Autodesk Inventor part; units mm, degrees
(part 2 of 3)
sketch "Эскиз5" plane through (0, 2, 0) normal (0, 1, 0) x (1, 0, 0)
  line L0 (-76.014, 34.2947) -> (-34.2947, 76.014) construction
  arc A0 (-34.2947, 76.014) -> (-34.2947, 83.085) centre (-37.8302, 79.5495) ccw construction
  line L1 (-34.2947, 83.085) -> (-38.3892, 87.1795) construction
  arc A1 (-37.7453, 90.4395) -> (-38.3892, 87.1795) centre (-36.975, 88.5938) ccw construction
  arc A2 (37.7453, 90.4395) -> (-37.7453, 90.4395) centre (0, 0) ccw construction
  arc A3 (38.3892, 87.1795) -> (37.7453, 90.4395) centre (36.975, 88.5938) ccw construction
  line L2 (38.3892, 87.1795) -> (34.2947, 83.085) construction
  arc A4 (34.2947, 83.085) -> (34.2947, 76.014) centre (37.8302, 79.5495) ccw construction
  line L3 (34.2947, 76.014) -> (76.014, 34.2947) construction
  arc A5 (48.6481, 93.0503) -> (-48.6481, 93.0503) centre (0, 0) ccw construction
  arc A6 (-48.6481, 93.0503) -> (-49.3795, 88.2704) centre (-47.2582, 90.3917) ccw construction
  line L4 (-49.3795, 88.2704) -> (-46.3155, 85.2064) construction
  arc A7 (-46.3155, 73.8927) -> (-46.3155, 85.2064) centre (-51.9723, 79.5495) ccw construction
  line L5 (-46.3155, 73.8927) -> (-73.8927, 46.3155) construction
  arc A8 (-85.2064, 46.3155) -> (-73.8927, 46.3155) centre (-79.5495, 51.9723) ccw construction
  line L6 (-85.2064, 46.3155) -> (-88.2704, 49.3795) construction
  arc A9 (-88.2704, 49.3795) -> (-93.0503, 48.6481) centre (-90.3917, 47.2582) ccw construction
  arc A10 (-93.0503, 48.6481) -> (-93.0503, -48.6481) centre (0, 0) ccw construction
  arc A11 (-93.0503, -48.6481) -> (-88.2704, -49.3795) centre (-90.3917, -47.2582) ccw construction
  line L7 (-88.2704, -49.3795) -> (-85.2064, -46.3155) construction
  arc A12 (-73.8927, -46.3155) -> (-85.2064, -46.3155) centre (-79.5495, -51.9723) ccw construction
  line L8 (-73.8927, -46.3155) -> (-46.3155, -73.8927) construction
  arc A13 (-46.3155, -85.2064) -> (-46.3155, -73.8927) centre (-51.9723, -79.5495) ccw construction
  line L9 (-46.3155, -85.2064) -> (-49.3795, -88.2704) construction
  arc A14 (-49.3795, -88.2704) -> (-48.6481, -93.0503) centre (-47.2582, -90.3917) ccw construction
  arc A15 (-48.6481, -93.0503) -> (-45.42, -94.668) centre (0, 0) ccw construction
  arc A16 (-45.42, -94.668) -> (-43.0355, -94.1655) centre (-44.5548, -92.8648) ccw construction
  line L10 (-43.0355, -94.1655) -> (-18.3802, -65.3664) construction
  arc A17 (-17.477, -64.7643) -> (-18.3802, -65.3664) centre (-16.8609, -66.6671) ccw construction
  line L11 (-17.477, -64.7643) -> (-0.6161, -59.3045) construction
  arc A18 (0.6161, -59.3045) -> (-0.6161, -59.3045) centre (0, -61.2072) ccw construction
  line L12 (0.6161, -59.3045) -> (17.477, -64.7643) construction
  arc A19 (18.3802, -65.3664) -> (17.477, -64.7643) centre (16.8609, -66.6671) ccw construction
  line L13 (18.3802, -65.3664) -> (43.0355, -94.1655) construction
  arc A20 (43.0355, -94.1655) -> (45.42, -94.668) centre (44.5548, -92.8648) ccw construction
  arc A21 (45.42, -94.668) -> (48.6481, -93.0503) centre (0, 0) ccw construction
  arc A22 (48.6481, -93.0503) -> (49.3795, -88.2704) centre (47.2582, -90.3917) ccw construction
  line L14 (49.3795, -88.2704) -> (46.3155, -85.2064) construction
  arc A23 (46.3155, -73.8927) -> (46.3155, -85.2064) centre (51.9723, -79.5495) ccw construction
  line L15 (46.3155, -73.8927) -> (73.8927, -46.3155) construction
  arc A24 (85.2064, -46.3155) -> (73.8927, -46.3155) centre (79.5495, -51.9723) ccw construction
  line L16 (85.2064, -46.3155) -> (88.2704, -49.3795) construction
  arc A25 (88.2704, -49.3795) -> (93.0503, -48.6481) centre (90.3917, -47.2582) ccw construction
  arc A26 (93.0503, -48.6481) -> (93.0503, 48.6481) centre (0, 0) ccw construction
  arc A27 (93.0503, 48.6481) -> (88.2704, 49.3795) centre (90.3917, 47.2582) ccw construction
  line L17 (88.2704, 49.3795) -> (85.2064, 46.3155) construction
  arc A28 (73.8927, 46.3155) -> (85.2064, 46.3155) centre (79.5495, 51.9723) ccw construction
  line L18 (73.8927, 46.3155) -> (46.3155, 73.8927) construction
  arc A29 (46.3155, 85.2064) -> (46.3155, 73.8927) centre (51.9723, 79.5495) ccw construction
  line L19 (46.3155, 85.2064) -> (49.3795, 88.2704) construction
  arc A30 (49.3795, 88.2704) -> (48.6481, 93.0503) centre (47.2582, 90.3917) ccw construction
  arc A31 (76.014, 34.2947) -> (83.085, 34.2947) centre (79.5495, 37.8302) ccw construction
  line L20 (83.085, 34.2947) -> (87.1795, 38.3892) construction
  arc A32 (90.4395, 37.7453) -> (87.1795, 38.3892) centre (88.5938, 36.975) ccw construction
  arc A33 (90.4395, -37.7453) -> (90.4395, 37.7453) centre (0, 0) ccw construction
  arc A34 (87.1795, -38.3892) -> (90.4395, -37.7453) centre (88.5938, -36.975) ccw construction
  line L21 (87.1795, -38.3892) -> (83.085, -34.2947) construction
  arc A35 (83.085, -34.2947) -> (76.014, -34.2947) centre (79.5495, -37.8302) ccw construction
  line L22 (76.014, -34.2947) -> (37.1244, -73.1843) construction
  line L23 (-37.1244, -73.1843) -> (-76.014, -34.2947) construction
  arc A36 (-76.014, -34.2947) -> (-83.085, -34.2947) centre (-79.5495, -37.8302) ccw construction
  line L24 (-83.085, -34.2947) -> (-87.1795, -38.3892) construction
  arc A37 (-90.4395, -37.7453) -> (-87.1795, -38.3892) centre (-88.5938, -36.975) ccw construction
  arc A38 (-90.4395, 37.7453) -> (-90.4395, -37.7453) centre (0, 0) ccw construction
  arc A39 (-87.1795, 38.3892) -> (-90.4395, 37.7453) centre (-88.5938, 36.975) ccw construction
  line L25 (-87.1795, 38.3892) -> (-83.085, 34.2947) construction
  arc A40 (-83.085, 34.2947) -> (-76.014, 34.2947) centre (-79.5495, 37.8302) ccw construction
  arc A41 (34.1909, -73.0707) -> (37.1244, -73.1843) centre (35.7102, -71.7701) ccw construction
  line L26 (34.1909, -73.0707) -> (25.4187, -62.8242) construction
  arc A42 (24.842, -61.8893) -> (25.4187, -62.8242) centre (28.1154, -60.5155) ccw construction
  line L27 (24.842, -61.8893) -> (23.8313, -59.4808) construction
  arc A43 (23.8313, -59.4808) -> (21.0049, -57.3328) centre (20.5578, -60.8546) ccw construction
  line L28 (21.0049, -57.3328) -> (15.1585, -56.5907) construction
  arc A44 (14.5119, -56.4463) -> (15.1585, -56.5907) centre (15.6055, -53.069) ccw construction
  line L29 (14.5119, -56.4463) -> (0.6161, -51.9466) construction
  arc A45 (0.6161, -51.9466) -> (-0.6161, -51.9466) centre (0, -53.8493) ccw construction
  line L30 (-0.6161, -51.9466) -> (-14.5119, -56.4463) construction
  arc A46 (-15.1585, -56.5907) -> (-14.5119, -56.4463) centre (-15.6055, -53.069) ccw construction
  line L31 (-15.1585, -56.5907) -> (-21.0049, -57.3328) construction
  arc A47 (-21.0049, -57.3328) -> (-23.8313, -59.4808) centre (-20.5578, -60.8546) ccw construction
  line L32 (-23.8313, -59.4808) -> (-24.842, -61.8893) construction
  arc A48 (-25.4187, -62.8242) -> (-24.842, -61.8893) centre (-28.1154, -60.5155) ccw construction
  line L33 (-25.4187, -62.8242) -> (-34.1909, -73.0707) construction
  arc A49 (-37.1244, -73.1843) -> (-34.1909, -73.0707) centre (-35.7102, -71.7701) ccw construction
  circle A50 centre (-37.8302, 79.5495) radius 1.6 construction
  circle A51 centre (-79.5495, 37.8302) radius 1.6 construction
  circle A52 centre (-79.5495, -37.8302) radius 1.6 construction
  circle A53 centre (79.5495, -37.8302) radius 1.6 construction
  circle A54 centre (37.8302, 79.5495) radius 1.6 construction
  circle A55 centre (79.5495, 37.8302) radius 1.6 construction
  circle A56 centre (-20.5578, -60.8546) radius 1.55 construction
  circle A57 centre (20.5578, -60.8546) radius 1.55 construction
  circle A58 centre (37.8302, -79.5495) radius 1.6 construction
  circle A59 centre (-37.8302, -79.5495) radius 1.6 construction
  circle A60 centre (0, -40) radius 1.6
  line L34 (0, -40.1335) -> (0, 0) construction
  arc A61 (0, -36) -> (-3.6492, -38.362) centre (0, -40) ccw
  line L35 (19.2746, -40.1335) -> (6.3862, -40.1335) construction
  line L36 (19.2746, -40.1335) -> (-19.2746, -40.1335) construction
  line L37 (-6.3862, -40.1335) -> (-19.2746, -40.1335) construction
  arc A62 (3.6492, -38.362) -> (0, -36) centre (0, -40) ccw
  arc A63 (-3.9978, -40.1335) -> (3.9978, -40.1335) centre (0, -40) ccw construction
  arc A64 (3.6492, -38.362) -> (6.3862, -40.1335) centre (6.3862, -37.1335) ccw
  arc A65 (-6.3862, -40.1335) -> (-3.6492, -38.362) centre (-6.3862, -37.1335) ccw
  line L38 (6.3862, -40.1335) -> (3.8373, -44.953)
  line L39 (3.8373, -44.953) -> (-3.2661, -45.2784)
  line L40 (-3.2661, -45.2784) -> (-6.3862, -40.1335)
  dimension "d100" = 3.2
  dimension "d101" = 40
  dimension "d103" = 3
  dimension "d104" = 4
  constraints: 12 end point, 12 point on circle, 6 centre point, 6 point on line, 4 tangent, 1 coincident, 1 equal radius, 1 vertical
  measures "d100" diameter of A60
  measures "d101" distance of point (0, 0) A60.centre
  measures "d103" radius of A64
  measures "d104" radius of A63
ref_plane "РабПлоскость8" through (0, 2, 0) normal (0, 1, 0) x (1, 0, 0)
sketch "Эскиз6" plane through (0, 2, 0) normal (0, 1, 0) x (1, 0, 0)
  line L0 (-76.014, 34.2947) -> (-34.2947, 76.014) construction
  arc A0 (-34.2947, 76.014) -> (-34.2947, 83.085) centre (-37.8302, 79.5495) ccw construction
  line L1 (-34.2947, 83.085) -> (-38.3892, 87.1795) construction
  arc A1 (-37.7453, 90.4395) -> (-38.3892, 87.1795) centre (-36.975, 88.5938) ccw construction
  arc A2 (37.7453, 90.4395) -> (-37.7453, 90.4395) centre (0, 0) ccw construction
  arc A3 (38.3892, 87.1795) -> (37.7453, 90.4395) centre (36.975, 88.5938) ccw construction
  line L2 (38.3892, 87.1795) -> (34.2947, 83.085) construction
  arc A4 (34.2947, 83.085) -> (34.2947, 76.014) centre (37.8302, 79.5495) ccw construction
  line L3 (34.2947, 76.014) -> (76.014, 34.2947) construction
  arc A5 (48.6481, 93.0503) -> (-48.6481, 93.0503) centre (0, 0) ccw construction
  arc A6 (-48.6481, 93.0503) -> (-49.3795, 88.2704) centre (-47.2582, 90.3917) ccw construction
  line L4 (-49.3795, 88.2704) -> (-46.3155, 85.2064) construction
  arc A7 (-46.3155, 73.8927) -> (-46.3155, 85.2064) centre (-51.9723, 79.5495) ccw construction
  line L5 (-46.3155, 73.8927) -> (-73.8927, 46.3155) construction
  arc A8 (-85.2064, 46.3155) -> (-73.8927, 46.3155) centre (-79.5495, 51.9723) ccw construction
  line L6 (-85.2064, 46.3155) -> (-88.2704, 49.3795) construction
  arc A9 (-88.2704, 49.3795) -> (-93.0503, 48.6481) centre (-90.3917, 47.2582) ccw construction
  arc A10 (-93.0503, 48.6481) -> (-93.0503, -48.6481) centre (0, 0) ccw construction
  arc A11 (-93.0503, -48.6481) -> (-88.2704, -49.3795) centre (-90.3917, -47.2582) ccw construction
  line L7 (-88.2704, -49.3795) -> (-85.2064, -46.3155) construction
  arc A12 (-73.8927, -46.3155) -> (-85.2064, -46.3155) centre (-79.5495, -51.9723) ccw construction
  line L8 (-73.8927, -46.3155) -> (-46.3155, -73.8927) construction
  arc A13 (-46.3155, -85.2064) -> (-46.3155, -73.8927) centre (-51.9723, -79.5495) ccw construction
  line L9 (-46.3155, -85.2064) -> (-49.3795, -88.2704) construction
  arc A14 (-49.3795, -88.2704) -> (-48.6481, -93.0503) centre (-47.2582, -90.3917) ccw construction
  arc A15 (-48.6481, -93.0503) -> (-45.42, -94.668) centre (0, 0) ccw construction
  arc A16 (-45.42, -94.668) -> (-43.0355, -94.1655) centre (-44.5548, -92.8648) ccw construction
  line L10 (-43.0355, -94.1655) -> (-18.3802, -65.3664) construction
  arc A17 (-17.477, -64.7643) -> (-18.3802, -65.3664) centre (-16.8609, -66.6671) ccw construction
  line L11 (-17.477, -64.7643) -> (-0.6161, -59.3045) construction
  arc A18 (0.6161, -59.3045) -> (-0.6161, -59.3045) centre (0, -61.2072) ccw construction
  line L12 (0.6161, -59.3045) -> (17.477, -64.7643) construction
  arc A19 (18.3802, -65.3664) -> (17.477, -64.7643) centre (16.8609, -66.6671) ccw construction
  line L13 (18.3802, -65.3664) -> (43.0355, -94.1655) construction
  arc A20 (43.0355, -94.1655) -> (45.42, -94.668) centre (44.5548, -92.8648) ccw construction
  arc A21 (45.42, -94.668) -> (48.6481, -93.0503) centre (0, 0) ccw construction
  arc A22 (48.6481, -93.0503) -> (49.3795, -88.2704) centre (47.2582, -90.3917) ccw construction
  line L14 (49.3795, -88.2704) -> (46.3155, -85.2064) construction
  arc A23 (46.3155, -73.8927) -> (46.3155, -85.2064) centre (51.9723, -79.5495) ccw construction
  line L15 (46.3155, -73.8927) -> (73.8927, -46.3155) construction
  arc A24 (85.2064, -46.3155) -> (73.8927, -46.3155) centre (79.5495, -51.9723) ccw construction
  line L16 (85.2064, -46.3155) -> (88.2704, -49.3795) construction
  arc A25 (88.2704, -49.3795) -> (93.0503, -48.6481) centre (90.3917, -47.2582) ccw construction
  arc A26 (93.0503, -48.6481) -> (93.0503, 48.6481) centre (0, 0) ccw construction
  arc A27 (93.0503, 48.6481) -> (88.2704, 49.3795) centre (90.3917, 47.2582) ccw construction
  line L17 (88.2704, 49.3795) -> (85.2064, 46.3155) construction
  arc A28 (73.8927, 46.3155) -> (85.2064, 46.3155) centre (79.5495, 51.9723) ccw construction
  line L18 (73.8927, 46.3155) -> (46.3155, 73.8927) construction
  arc A29 (46.3155, 85.2064) -> (46.3155, 73.8927) centre (51.9723, 79.5495) ccw construction
  line L19 (46.3155, 85.2064) -> (49.3795, 88.2704) construction
  arc A30 (49.3795, 88.2704) -> (48.6481, 93.0503) centre (47.2582, 90.3917) ccw construction
  arc A31 (76.014, 34.2947) -> (83.085, 34.2947) centre (79.5495, 37.8302) ccw construction
  line L20 (83.085, 34.2947) -> (87.1795, 38.3892) construction
  arc A32 (90.4395, 37.7453) -> (87.1795, 38.3892) centre (88.5938, 36.975) ccw construction
  arc A33 (90.4395, -37.7453) -> (90.4395, 37.7453) centre (0, 0) ccw construction
  arc A34 (87.1795, -38.3892) -> (90.4395, -37.7453) centre (88.5938, -36.975) ccw construction
  line L21 (87.1795, -38.3892) -> (83.085, -34.2947) construction
  arc A35 (83.085, -34.2947) -> (76.014, -34.2947) centre (79.5495, -37.8302) ccw construction
  line L22 (76.014, -34.2947) -> (37.1244, -73.1843) construction
  line L23 (-37.1244, -73.1843) -> (-76.014, -34.2947) construction
  arc A36 (-76.014, -34.2947) -> (-83.085, -34.2947) centre (-79.5495, -37.8302) ccw construction
  line L24 (-83.085, -34.2947) -> (-87.1795, -38.3892) construction
  arc A37 (-90.4395, -37.7453) -> (-87.1795, -38.3892) centre (-88.5938, -36.975) ccw construction
  arc A38 (-90.4395, 37.7453) -> (-90.4395, -37.7453) centre (0, 0) ccw construction
  arc A39 (-87.1795, 38.3892) -> (-90.4395, 37.7453) centre (-88.5938, 36.975) ccw construction
  line L25 (-87.1795, 38.3892) -> (-83.085, 34.2947) construction
  arc A40 (-83.085, 34.2947) -> (-76.014, 34.2947) centre (-79.5495, 37.8302) ccw construction
  arc A41 (34.1909, -73.0707) -> (37.1244, -73.1843) centre (35.7102, -71.7701) ccw construction
  line L26 (34.1909, -73.0707) -> (25.4187, -62.8242) construction
  arc A42 (24.842, -61.8893) -> (25.4187, -62.8242) centre (28.1154, -60.5155) ccw construction
  line L27 (24.842, -61.8893) -> (23.8313, -59.4808) construction
  arc A43 (23.8313, -59.4808) -> (21.0049, -57.3328) centre (20.5578, -60.8546) ccw construction
  line L28 (21.0049, -57.3328) -> (15.1585, -56.5907) construction
  arc A44 (14.5119, -56.4463) -> (15.1585, -56.5907) centre (15.6055, -53.069) ccw construction
  line L29 (14.5119, -56.4463) -> (0.6161, -51.9466) construction
  arc A45 (0.6161, -51.9466) -> (-0.6161, -51.9466) centre (0, -53.8493) ccw construction
  line L30 (-0.6161, -51.9466) -> (-14.5119, -56.4463) construction
  arc A46 (-15.1585, -56.5907) -> (-14.5119, -56.4463) centre (-15.6055, -53.069) ccw construction
  line L31 (-15.1585, -56.5907) -> (-21.0049, -57.3328) construction
  arc A47 (-21.0049, -57.3328) -> (-23.8313, -59.4808) centre (-20.5578, -60.8546) ccw construction
  line L32 (-23.8313, -59.4808) -> (-24.842, -61.8893) construction
  arc A48 (-25.4187, -62.8242) -> (-24.842, -61.8893) centre (-28.1154, -60.5155) ccw construction
  line L33 (-25.4187, -62.8242) -> (-34.1909, -73.0707) construction
  arc A49 (-37.1244, -73.1843) -> (-34.1909, -73.0707) centre (-35.7102, -71.7701) ccw construction
  circle A50 centre (-37.8302, 79.5495) radius 1.6 construction
  circle A51 centre (-79.5495, 37.8302) radius 1.6 construction
  circle A52 centre (-79.5495, -37.8302) radius 1.6 construction
  circle A53 centre (79.5495, -37.8302) radius 1.6 construction
  circle A54 centre (37.8302, 79.5495) radius 1.6 construction
  circle A55 centre (79.5495, 37.8302) radius 1.6 construction
  circle A56 centre (-20.5578, -60.8546) radius 1.55 construction
  circle A57 centre (20.5578, -60.8546) radius 1.55 construction
  circle A58 centre (37.8302, -79.5495) radius 1.6 construction
  circle A59 centre (-37.8302, -79.5495) radius 1.6 construction
  line L34 (0, 0) -> (0, 105) construction
  arc A60 (48.6481, 93.0503) -> (-48.6481, 93.0503) centre (0, 0) ccw construction
  line L35 (-19.5, 5.5231) -> (19.5, 5.5231) construction
  line L36 (19.5, 5.5231) -> (19.5, 136.6901) construction
  line L37 (19.5, 136.6901) -> (-19.5, 136.6901) construction
  line L38 (-19.5, 136.6901) -> (-19.5, 5.5231) construction
  circle A61 centre (-24, 98.1071) radius 4 construction
  circle A62 centre (24, 98.1071) radius 4 construction
  arc A63 (-21.3158, 95.1414) -> (20.4598, 95.3292) centre (0, 0) ccw construction
  arc A64 (-23.5, 93.6349) -> (-20.4598, 95.3292) centre (-24, 98.1071) ccw
  line L39 (-23.5, 49.663) -> (-23.5, 93.6349)
  line L40 (-20, 47.2032) -> (-20, 95.4267)
  arc A65 (-19.0919, 46.6335) -> (-21.4454, 47.6084) centre (-21.9203, 43.1335) ccw
  line L41 (-21.4454, 47.6084) -> (-23.5, 49.663)
  line L42 (-21.6698, 47.1257) -> (-42.4264, 67.8823) construction
  line L43 (-42.4264, 67.8823) -> (-34.2947, 76.014) construction
  line L44 (-19.0919, 46.6335) -> (-6.5611, 46.6335)
  arc A66 (0, 41.5) -> (3.9366, 48.1801) centre (0, 46) ccw construction
  arc A67 (-4.4552, 46.6335) -> (0, 41.5) centre (0, 46) ccw construction
  arc A68 (-6.5611, 46.6335) -> (-3.9366, 48.1801) centre (-6.5611, 49.6335) ccw
  line L45 (-23.5, 49.663) -> (-42.0729, 68.2358) construction
  arc A69 (-18.5662, 46.1335) -> (-19.0919, 46.6335) centre (-21.9203, 43.1335) ccw construction
  arc A70 (-21.4454, 47.6084) -> (-18.5662, 46.1335) centre (-21.9203, 43.1335) ccw construction
  arc A71 (-25.858, 94.0086) -> (-23.5, 93.6349) centre (-24, 98.1071) ccw construction
  arc A72 (-20.4598, 95.3292) -> (-25.858, 94.0086) centre (-24, 98.1071) ccw construction
  arc A73 (-20.4598, 95.3292) -> (-21.3158, 95.1414) centre (0, 0) ccw construction
  arc A74 (20.4598, 95.3292) -> (23.5, 93.6349) centre (24, 98.1071) ccw
  line L46 (23.5, 49.663) -> (23.5, 93.6349)
  line L47 (20, 47.2032) -> (20, 95.4267)
  arc A75 (21.4454, 47.6084) -> (19.0919, 46.6335) centre (21.9203, 43.1335) ccw
  line L48 (21.4454, 47.6084) -> (23.5, 49.663)
  line L49 (19.0919, 46.6335) -> (6.5611, 46.6335)
  arc A76 (3.9366, 48.1801) -> (6.5611, 46.6335) centre (6.5611, 49.6335) ccw
  arc A77 (3.9366, 48.1801) -> (-3.9366, 48.1801) centre (0, 46) ccw
  arc A78 (20.4598, 95.3292) -> (-20.4598, 95.3292) centre (0, 0) ccw
  circle A79 centre (0, 46) radius 1.5
  dimension "d112" = 8
  dimension "d111" = 39
  dimension "d114" = 9
  dimension "d115" = 4
  dimension "d116" = 0.5
  dimension "d117" = 9
  dimension "d118" = 0.5
  dimension "d120" = 9
  dimension "d121" = 3
  dimension "d179" = 3
  constraints: 42 point on circle, 28 end point, 18 centre point, 13 symmetric about line, 4 parallel, 3 coincident, 3 point on line, 2 horizontal, 2 tangent, 2 vertical, 1 perpendicular, 8 other
  measures "d111" distance of L37.end L36.end
  measures "d114" diameter of A64
  measures "d115" distance between parallel lines of L38 L39
  measures "d116" distance between parallel lines of L38 L40
  measures "d117" diameter of A65
  measures "d118" distance between parallel lines of L42 L41
  measures "d120" diameter of A66
  measures "d121" radius of A68
  measures "d179" diameter of A79
extrude "Выдавливание9" add sketch "Эскиз6" along normal blind 1.85 and the other way blind 2 contours A64 A78 L40 A65 L41 L39 | A78 L47 A75 L49 A76 A77 A68 L44 A65 L40 | A78 A74 L46 L48 A75 L47
extrude "Выдавливание10" add sketch "Эскиз6" along normal blind 6.85 contours A64 A78 L40 A65 L41 L39 | A78 A74 L46 L48 A75 L47
ref_plane "РабПлоскость1" through (0, 8.85, 0) normal (0, 1, 0) x (1, 0, 0)
sketch "Эскиз7" plane through (0, 8.85, 0) normal (0, 1, 0) x (1, 0, 0)
  line L0 (-20, 95.4267) -> (-20, 47.2032) projected
  arc A0 (-19.0919, 46.6335) -> (-20, 47.2032) centre (-21.9203, 43.1335) ccw projected
  line L1 (-19.0919, 46.6335) -> (-6.5611, 46.6335) projected
  arc A1 (-6.5611, 46.6335) -> (-3.9366, 48.1801) centre (-6.5611, 49.6335) ccw construction
  arc A2 (3.9366, 48.1801) -> (-3.9366, 48.1801) centre (0, 46) ccw construction
  arc A3 (3.9366, 48.1801) -> (6.5611, 46.6335) centre (6.5611, 49.6335) ccw construction
  line L2 (6.5611, 46.6335) -> (19.0919, 46.6335) projected
  arc A4 (20, 47.2032) -> (19.0919, 46.6335) centre (21.9203, 43.1335) ccw projected
  line L3 (20, 47.2032) -> (20, 95.4267) projected
  arc A5 (20, 95.4267) -> (-20, 95.4267) centre (0, 0) ccw projected
  arc A6 (-20, 95.4267) -> (-20.4598, 95.3292) centre (0, 0) ccw projected
  arc A7 (-23.5, 93.6349) -> (-20.4598, 95.3292) centre (-24, 98.1071) ccw projected
  line L4 (-23.5, 93.6349) -> (-23.5, 49.663) projected
  line L5 (-23.5, 49.663) -> (-21.4454, 47.6084) projected
  arc A8 (-20, 47.2032) -> (-21.4454, 47.6084) centre (-21.9203, 43.1335) ccw projected
  line L6 (-20, 47.2032) -> (-20, 95.4267) projected
  arc A9 (20.4598, 95.3292) -> (20, 95.4267) centre (0, 0) ccw projected
  line L7 (20, 95.4267) -> (20, 47.2032) projected
  arc A10 (21.4454, 47.6084) -> (20, 47.2032) centre (21.9203, 43.1335) ccw projected
  line L8 (21.4454, 47.6084) -> (23.5, 49.663) projected
  line L9 (23.5, 49.663) -> (23.5, 93.6349) projected
  arc A11 (20.4598, 95.3292) -> (23.5, 93.6349) centre (24, 98.1071) ccw projected
  line L10 (18.2, 46.6335) -> (18.2, 95.7863)
  arc A12 (3.5768, 47.7906) -> (-3.5768, 47.7906) centre (0, 46) ccw construction
  line L11 (0, 46) -> (0, 97.5) construction
  line L12 (-18.2, 46.6335) -> (-18.2, 95.7863)
  point P0 (-20, 95.4267)
  point P1 (-20, 47.2032)
  dimension "d129" = 1.8
  constraints: 6 end point, 2 point on circle, 2 symmetric about line, 1 point on line, 1 vertical
  measures "d129" distance between parallel lines of L3 L10
extrude "Выдавливание11" add sketch "Эскиз7" along normal blind 5
chamfer "Фаска1" distance 1.8 angle 45 2 edges at (18.2, 8.85, -71.2099) (-18.2, 8.85, -71.2099)
fillet "Сопряжение1" radius 3 2 edges at (23.5, 13.85, -71.6489) (-23.5, 13.85, -71.6489)
fillet "Сопряжение2" radius 1 2 edges at (18.2, 13.85, -71.2099) (-18.2, 13.85, -71.2099)
ref_plane "РабПлоскость2" through (6.5611, 3.85, -46.6335) normal (0, 0, 1) x (1, 0, 0)
sketch "Эскиз8" plane through (6.5611, 3.85, -46.6335) normal (0, 0, 1) x (1, 0, 0)
  line L0 (-26.5611, 0) -> (-25.6529, 0) construction
  line L1 (-25.6529, 0) -> (-13.1221, 0) construction
  line L2 (-13.1221, 0) -> (-10.4977, 0) construction
  line L3 (-10.4977, 0) -> (-2.6244, 0) construction
  line L4 (-2.6244, 0) -> (0, 0) construction
  line L5 (0, 0) -> (12.5308, 0) construction
  line L6 (12.5308, 0) -> (13.4389, 0) construction
  line L7 (13.4389, 0) -> (-26.5611, 0) construction
  line L8 (-24.7611, 6.8) -> (-24.7611, 9) construction
  line L9 (-26.5611, 5) -> (-24.7611, 6.8) construction
  line L10 (-26.5611, 0) -> (-26.5611, 5) construction
  line L11 (13.4389, 0) -> (-26.5611, 0) construction
  line L12 (13.4389, 0) -> (13.4389, 5) construction
  line L13 (11.6389, 6.8) -> (13.4389, 5) construction
  line L14 (11.6389, 6.8) -> (11.6389, 9) construction
  line L15 (13.8987, 10) -> (12.6389, 10) construction
  line L16 (13.8987, -3.85) -> (13.8987, 10) construction
  line L17 (-27.0209, -3.85) -> (13.8987, -3.85) construction
  line L18 (-27.0209, -3.85) -> (-27.0209, 10) construction
  line L19 (-25.7611, 10) -> (-27.0209, 10) construction
  line L20 (-27.0209, 10) -> (-27.0611, 10) construction
  line L21 (-27.0209, -3.85) -> (-27.0209, 10) construction
  line L22 (-30.0611, -3.85) -> (-27.0209, -3.85) construction
  line L23 (-30.0611, -3.85) -> (-30.0611, 7) construction
  line L24 (16.9389, -3.85) -> (16.9389, 7) construction
  line L25 (13.8987, -3.85) -> (16.9389, -3.85) construction
  line L26 (13.8987, -3.85) -> (13.8987, 10) construction
  line L27 (13.9389, 10) -> (13.8987, 10) construction
  line L28 (-6.5611, -3.85) -> (-6.5611, 0) construction
  line L29 (-6.5611, -1.85) -> (-6.5611, 0.15) construction
  line L30 (-8.1611, -1.85) -> (-4.9611, -1.85) construction
  line L31 (-11.4446, 0.15) -> (-1.6776, 0.15) construction
  line L32 (-6.5611, -1.85) -> (-4.0611, -1.85) construction
  line L33 (-4.0611, -1.85) -> (-1.6776, 0.15) construction
  line L34 (-6.5611, -1.85) -> (-9.0611, -1.85) construction
  line L35 (-9.0611, -1.85) -> (-11.4446, 0.15) construction
  line L36 (-11.7325, 0) -> (-9.5278, -1.85)
  line L37 (-2.9842, -1.85) -> (-10.1379, -1.85) construction
  line L38 (-1.3896, 0) -> (-3.5943, -1.85)
  line L39 (-1.3896, 0) -> (-11.7325, 0)
  line L40 (13.4389, 0) -> (-26.5611, 0) projected
  line L41 (-9.5278, -1.85) -> (-3.5943, -1.85)
  dimension "d138" = 2
  dimension "d139" = 2.5
  dimension "d141" = 40
  dimension "d142" = 0.3
  constraints: 22 end point, 5 point on line, 4 symmetric about line, 3 midpoint, 2 collinear, 2 parallel, 1 horizontal, 5 other
  measures "d138" distance of L29.start L29.end
  measures "d139" distance of L29.start L32.end
  measures "d141" angle of L31 L33
  measures "d142" distance between parallel lines of L35 L36
extrude "Выдавливание12" cut sketch "Эскиз8" against normal mid plane 300
ref_plane "РабПлоскость9" through (0, 2, 0) normal (0, 1, 0) x (1, 0, 0)
sketch "Эскиз9" plane through (0, 2, 0) normal (0, 1, 0) x (1, 0, 0)
  line L0 (-20, 95.4267) -> (-20, 47.2032) construction
  line L1 (-20, 47.2032) -> (-20, 95.4267) construction
  line L2 (63.6396, 46.669) -> (43.8406, 26.8701) construction
  line L3 (20, 47.2032) -> (20, 95.4267) construction
  line L4 (20, 95.4267) -> (20, 47.2032) construction
  circle A0 centre (-24, 98.1071) radius 1.6 construction
  arc A1 (-25.8102, 94.5401) -> (-20.7476, 95.7786) centre (-24, 98.1071) ccw construction
  circle A2 centre (24, 98.1071) radius 1.6 construction
  arc A3 (20.7476, 95.7786) -> (25.8102, 94.5401) centre (24, 98.1071) ccw construction
  arc A4 (-27.022, 95.4865) -> (-25, 94.2341) centre (-24, 98.1071) ccw
  line L5 (-34.2947, 83.085) -> (-38.3892, 87.1795) construction
  line L6 (76.014, -34.2947) -> (37.1244, -73.1843) construction
  arc A5 (34.1909, -73.0707) -> (37.1244, -73.1843) centre (35.7102, -71.7701) ccw construction
  line L7 (34.1909, -73.0707) -> (25.4187, -62.8242) construction
  arc A6 (24.842, -61.8893) -> (25.4187, -62.8242) centre (28.1154, -60.5155) ccw construction
  line L8 (24.842, -61.8893) -> (23.8313, -59.4808) construction
  arc A7 (23.8313, -59.4808) -> (21.0049, -57.3328) centre (20.5578, -60.8546) ccw construction
  line L9 (21.0049, -57.3328) -> (15.1585, -56.5907) construction
  arc A8 (14.5119, -56.4463) -> (15.1585, -56.5907) centre (15.6055, -53.069) ccw construction
  line L10 (14.5119, -56.4463) -> (0.6161, -51.9466) construction
  arc A9 (0.6161, -51.9466) -> (-0.6161, -51.9466) centre (0, -53.8493) ccw construction
  line L11 (-0.6161, -51.9466) -> (-14.5119, -56.4463) construction
  arc A10 (-15.1585, -56.5907) -> (-14.5119, -56.4463) centre (-15.6055, -53.069) ccw construction
  line L12 (-15.1585, -56.5907) -> (-21.0049, -57.3328) construction
  arc A11 (-21.0049, -57.3328) -> (-23.8313, -59.4808) centre (-20.5578, -60.8546) ccw construction
  line L13 (-23.8313, -59.4808) -> (-24.842, -61.8893) construction
  arc A12 (-25.4187, -62.8242) -> (-24.842, -61.8893) centre (-28.1154, -60.5155) ccw construction
  line L14 (-25.4187, -62.8242) -> (-34.1909, -73.0707) construction
  arc A13 (-37.1244, -73.1843) -> (-34.1909, -73.0707) centre (-35.7102, -71.7701) ccw construction
  line L15 (-37.1244, -73.1843) -> (-76.014, -34.2947) construction
  line L16 (-76.014, 34.2947) -> (-34.2947, 76.014) construction
  arc A14 (-34.2947, 76.014) -> (-34.2947, 83.085) centre (-37.8302, 79.5495) ccw construction
  line L17 (-34.2947, 83.085) -> (-38.3892, 87.1795) construction
  arc A15 (-37.7453, 90.4395) -> (-38.3892, 87.1795) centre (-36.975, 88.5938) ccw construction
  arc A16 (37.7453, 90.4395) -> (-37.7453, 90.4395) centre (0, 0) ccw construction
  arc A17 (38.3892, 87.1795) -> (37.7453, 90.4395) centre (36.975, 88.5938) ccw construction
  line L18 (38.3892, 87.1795) -> (34.2947, 83.085) construction
  arc A18 (34.2947, 83.085) -> (34.2947, 76.014) centre (37.8302, 79.5495) ccw construction
  line L19 (34.2947, 76.014) -> (76.014, 34.2947) construction
  arc A19 (76.014, 34.2947) -> (83.085, 34.2947) centre (79.5495, 37.8302) ccw construction
  line L20 (83.085, 34.2947) -> (87.1795, 38.3892) construction
  arc A20 (90.4395, 37.7453) -> (87.1795, 38.3892) centre (88.5938, 36.975) ccw construction
  arc A21 (90.4395, -37.7453) -> (90.4395, 37.7453) centre (0, 0) ccw construction
  arc A22 (87.1795, -38.3892) -> (90.4395, -37.7453) centre (88.5938, -36.975) ccw construction
  line L21 (87.1795, -38.3892) -> (83.085, -34.2947) construction
  arc A23 (83.085, -34.2947) -> (76.014, -34.2947) centre (79.5495, -37.8302) ccw construction
  circle A24 centre (79.5495, -37.8302) radius 1.6 construction
  circle A25 centre (37.8302, 79.5495) radius 1.6 construction
  circle A26 centre (79.5495, 37.8302) radius 1.6 construction
  circle A27 centre (20.5578, -60.8546) radius 1.55 construction
  circle A28 centre (37.8302, -79.5495) radius 1.6 construction
  arc A29 (48.6481, 93.0503) -> (-48.6481, 93.0503) centre (0, 0) ccw construction
  arc A30 (-48.6481, 93.0503) -> (-49.3795, 88.2704) centre (-47.2582, 90.3917) ccw construction
  line L22 (-49.3795, 88.2704) -> (-46.3155, 85.2064) construction
  arc A31 (-46.3155, 73.8927) -> (-46.3155, 85.2064) centre (-51.9723, 79.5495) ccw construction
  line L23 (-46.3155, 73.8927) -> (-73.8927, 46.3155) construction
  arc A32 (-85.2064, 46.3155) -> (-73.8927, 46.3155) centre (-79.5495, 51.9723) ccw construction
  line L24 (-85.2064, 46.3155) -> (-88.2704, 49.3795) construction
  arc A33 (-88.2704, 49.3795) -> (-93.0503, 48.6481) centre (-90.3917, 47.2582) ccw construction
  arc A34 (-93.0503, 48.6481) -> (-93.0503, -48.6481) centre (0, 0) ccw construction
  arc A35 (-93.0503, -48.6481) -> (-88.2704, -49.3795) centre (-90.3917, -47.2582) ccw construction
  line L25 (-88.2704, -49.3795) -> (-85.2064, -46.3155) construction
  arc A36 (-73.8927, -46.3155) -> (-85.2064, -46.3155) centre (-79.5495, -51.9723) ccw construction
  line L26 (-73.8927, -46.3155) -> (-46.3155, -73.8927) construction
  arc A37 (-46.3155, -85.2064) -> (-46.3155, -73.8927) centre (-51.9723, -79.5495) ccw construction
  line L27 (-46.3155, -85.2064) -> (-49.3795, -88.2704) construction
  arc A38 (-49.3795, -88.2704) -> (-48.6481, -93.0503) centre (-47.2582, -90.3917) ccw construction
  arc A39 (-48.6481, -93.0503) -> (-45.42, -94.668) centre (0, 0) ccw construction
  arc A40 (-45.42, -94.668) -> (-43.0355, -94.1655) centre (-44.5548, -92.8648) ccw construction
  line L28 (-43.0355, -94.1655) -> (-18.3802, -65.3664) construction
  arc A41 (-17.477, -64.7643) -> (-18.3802, -65.3664) centre (-16.8609, -66.6671) ccw construction
  line L29 (-17.477, -64.7643) -> (-0.6161, -59.3045) construction
  arc A42 (0.6161, -59.3045) -> (-0.6161, -59.3045) centre (0, -61.2072) ccw construction
  line L30 (0.6161, -59.3045) -> (17.477, -64.7643) construction
  arc A43 (18.3802, -65.3664) -> (17.477, -64.7643) centre (16.8609, -66.6671) ccw construction
  line L31 (18.3802, -65.3664) -> (43.0355, -94.1655) construction
  arc A44 (43.0355, -94.1655) -> (45.42, -94.668) centre (44.5548, -92.8648) ccw construction
  arc A45 (45.42, -94.668) -> (48.6481, -93.0503) centre (0, 0) ccw construction
  arc A46 (48.6481, -93.0503) -> (49.3795, -88.2704) centre (47.2582, -90.3917) ccw construction
  line L32 (49.3795, -88.2704) -> (46.3155, -85.2064) construction
  arc A47 (46.3155, -73.8927) -> (46.3155, -85.2064) centre (51.9723, -79.5495) ccw construction
  line L33 (46.3155, -73.8927) -> (73.8927, -46.3155) construction
  arc A48 (85.2064, -46.3155) -> (73.8927, -46.3155) centre (79.5495, -51.9723) ccw construction
  line L34 (85.2064, -46.3155) -> (88.2704, -49.3795) construction
  arc A49 (88.2704, -49.3795) -> (93.0503, -48.6481) centre (90.3917, -47.2582) ccw construction
  arc A50 (93.0503, -48.6481) -> (93.0503, 48.6481) centre (0, 0) ccw construction
  arc A51 (93.0503, 48.6481) -> (88.2704, 49.3795) centre (90.3917, 47.2582) ccw construction
  line L35 (88.2704, 49.3795) -> (85.2064, 46.3155) construction
  arc A52 (73.8927, 46.3155) -> (85.2064, 46.3155) centre (79.5495, 51.9723) ccw construction
  line L36 (73.8927, 46.3155) -> (46.3155, 73.8927) construction
  arc A53 (46.3155, 85.2064) -> (46.3155, 73.8927) centre (51.9723, 79.5495) ccw construction
  line L37 (46.3155, 85.2064) -> (49.3795, 88.2704) construction
  arc A54 (49.3795, 88.2704) -> (48.6481, 93.0503) centre (47.2582, 90.3917) ccw construction
  arc A55 (-76.014, -34.2947) -> (-83.085, -34.2947) centre (-79.5495, -37.8302) ccw construction
  line L38 (-83.085, -34.2947) -> (-87.1795, -38.3892) construction
  arc A56 (-90.4395, -37.7453) -> (-87.1795, -38.3892) centre (-88.5938, -36.975) ccw construction
  arc A57 (-90.4395, 37.7453) -> (-90.4395, -37.7453) centre (0, 0) ccw construction
  arc A58 (-87.1795, 38.3892) -> (-90.4395, 37.7453) centre (-88.5938, 36.975) ccw construction
  line L39 (-87.1795, 38.3892) -> (-83.085, 34.2947) construction
  arc A59 (-83.085, 34.2947) -> (-76.014, 34.2947) centre (-79.5495, 37.8302) ccw construction
  circle A60 centre (-37.8302, 79.5495) radius 1.6 construction
  circle A61 centre (-79.5495, 37.8302) radius 1.6 construction
  circle A62 centre (-79.5495, -37.8302) radius 1.6 construction
  circle A63 centre (-20.5578, -60.8546) radius 1.55 construction
  circle A64 centre (-37.8302, -79.5495) radius 1.6 construction
  line L40 (-20, 47.2032) -> (-20, 101.8577) construction
  arc A65 (48.6481, 93.0503) -> (-48.6481, 93.0503) centre (0, 0) ccw construction
  line L41 (-34.2947, 83.085) -> (-38.3892, 87.1795) construction
  line L42 (-34.2947, 83.085) -> (-45.7288, 94.5192) construction
  arc A66 (-48.6481, 93.0503) -> (-20, 103.0776) centre (0, 0) ccw construction
  arc A67 (-45.7288, 94.5192) -> (-48.6481, 93.0503) centre (0, 0) ccw construction
  arc A68 (-42.7269, 91.5173) -> (-27.8658, 97.0798) centre (0, 0) ccw construction
  line L43 (-34.7466, 84.2441) -> (-42.2438, 91.7413) construction
  line L44 (-45.2513, 94.7487) -> (-48.7043, 98.2018) construction
  line L45 (-42.7346, 92.2321) -> (-44.244, 93.7415)
  arc A69 (-42.2438, 91.7413) -> (-42.7269, 91.5173) centre (0, 0) ccw construction
  arc A70 (-45.2513, 94.7487) -> (-45.7288, 94.5192) centre (0, 0) ccw construction
  arc A71 (-43.9555, 95.3568) -> (-44.244, 93.7415) centre (-43.5369, 94.4486) ccw
  arc A72 (-42.7346, 92.2321) -> (-41.6155, 92.028) centre (-42.0275, 92.9392) ccw
  arc A73 (-30.1851, 96.3839) -> (-41.6155, 92.028) centre (0, 0) ccw
  arc A74 (-24.9505, 101.9925) -> (-27.8658, 97.0798) centre (-24, 98.1071) ccw
  arc A75 (-27.022, 95.4865) -> (-30.1851, 96.3839) centre (-29.2885, 93.521) ccw
  arc A76 (-21.2019, 102.8371) -> (-43.9555, 95.3568) centre (0, 0) ccw construction
  arc A77 (-20, 101.8577) -> (-21.2019, 102.8371) centre (-21, 101.8577) ccw
  line L46 (-20, 95.4267) -> (-20, 98.1071)
  arc A78 (-23.5, 93.6349) -> (-20.4598, 95.3292) centre (-24, 98.1071) ccw construction
  line L47 (-23.5, 49.663) -> (-23.5, 93.6349) construction
  line L48 (-23.5, 49.663) -> (-23.5, 92.2976) construction
  arc A79 (-23.5, 92.2976) -> (-25, 94.2341) centre (-25.5, 92.2976) ccw
  line L49 (-20, 98.1071) -> (-20, 101.8577)
  arc A80 (-21.2019, 102.8371) -> (-43.9555, 95.3568) centre (0, 0) ccw
  line L50 (0, 46) -> (0, 105) construction
  arc A81 (44.244, 93.7415) -> (43.9555, 95.3568) centre (43.5369, 94.4486) ccw
  arc A82 (41.6155, 92.028) -> (42.7346, 92.2321) centre (42.0275, 92.9392) ccw
  arc A83 (41.6155, 92.028) -> (30.1851, 96.3839) centre (0, 0) ccw
  arc A84 (30.1851, 96.3839) -> (27.022, 95.4865) centre (29.2885, 93.521) ccw
  arc A85 (21.2019, 102.8371) -> (20, 101.8577) centre (21, 101.8577) ccw
  line L51 (20, 95.4267) -> (20, 98.1071)
  arc A86 (25, 94.2341) -> (23.5, 92.2976) centre (25.5, 92.2976) ccw
  line L52 (20, 98.1071) -> (20, 101.8577)
  arc A87 (43.9555, 95.3568) -> (21.2019, 102.8371) centre (0, 0) ccw
  line L53 (42.7346, 92.2321) -> (44.244, 93.7415)
  arc A88 (-20, 99) -> (-30.1851, 96.3839) centre (0, 0) ccw
  arc A89 (30.1851, 96.3839) -> (20, 99) centre (0, 0) ccw
  line L54 (-20, 95.4267) -> (-20, 47.2032) projected
  line L55 (-23.5, 92.2976) -> (-20, 95.4267)
  arc A90 (25, 94.2341) -> (27.022, 95.4865) centre (24, 98.1071) ccw
  line L56 (23.5, 92.2976) -> (20, 95.4267)
  arc A91 (3.9495, 46.6335) -> (-3.9495, 46.6335) centre (0, 46) ccw
  line L57 (-6.5611, 46.6335) -> (-19.0919, 46.6335) projected
  line L58 (-19.0919, 46.6335) -> (-6.5878, 46.6335)
  line L59 (187.2372, 46.6335) -> (-186.873, 46.6335) projected
  arc A92 (-3.7645, 44.6477) -> (3.9495, 46.6335) centre (0, 46) ccw
  arc A93 (-3.7645, 44.6477) -> (-6.5878, 46.6335) centre (-6.5878, 43.6335) ccw
  arc A94 (6.5878, 46.6335) -> (3.7645, 44.6477) centre (6.5878, 43.6335) ccw
  arc A95 (3.9366, 48.1801) -> (6.5611, 46.6335) centre (6.5611, 49.6335) ccw projected
  line L60 (6.5611, 46.6335) -> (6.5878, 51)
  line L61 (6.5878, 51) -> (-6.2595, 51)
  arc A96 (-6.5611, 46.6335) -> (-3.9366, 48.1801) centre (-6.5611, 49.6335) ccw projected
  line L62 (-6.2595, 51) -> (-6.5611, 46.6335)
  arc A97 (3.9366, 48.1801) -> (-3.9366, 48.1801) centre (0, 46) ccw projected
  arc A98 (3.5768, 47.7906) -> (-3.5768, 47.7906) centre (0, 46) ccw projected
  arc A99 (-2.9667, 97.4549) -> (-5.1715, 97.3628) centre (0, 0) ccw construction
  line L63 (-5.1715, 46.9748) -> (-5.1715, 97.3628) construction
  arc A100 (-5.1715, 46.9748) -> (-3.9366, 48.1801) centre (-6.5611, 49.6335) ccw construction
  arc A101 (-2.9667, 49.3836) -> (-3.9366, 48.1801) centre (0, 46) ccw construction
  line L64 (-2.9667, 97.4549) -> (-2.9667, 49.3836) construction
  arc A102 (5.1715, 97.3628) -> (2.9667, 97.4549) centre (0, 0) ccw construction
  line L65 (2.9667, 49.3836) -> (2.9667, 97.4549) construction
  arc A103 (3.9366, 48.1801) -> (2.9667, 49.3836) centre (0, 46) ccw construction
  arc A104 (3.9366, 48.1801) -> (5.1715, 46.9748) centre (6.5611, 49.6335) ccw construction
  line L66 (5.1715, 97.3628) -> (5.1715, 46.9748) construction
  circle A105 centre (0, 0) radius 98 construction
  circle A106 centre (0, 46) radius 1.55
  point P0 (-23.5, 94.1385)
  point P1 (20, 99)
  point P2 (3.7645, 44.6477)
  point P3 (1.4146, 46.6335)
  point P4 (-1.4146, 46.6335)
  dimension "d147" = 8
  dimension "d148" = 4
  dimension "d149" = 0.5
  dimension "d150" = 1
  dimension "d151" = 3
  dimension "d152" = 1
  dimension "d153" = 2
  dimension "d161" = 8
  dimension "d162" = 3
  dimension "d165" = 5
  dimension "d169" = 196
  dimension "d180" = 3.1
  constraints: 75 point on circle, 36 end point, 31 centre point, 22 symmetric about line, 12 tangent, 10 point on line, 9 coincident, 4 collinear, 4 parallel, 2 equal radius, 2 vertical, 10 other
  measures "d147" diameter of A4
  measures "d148" radial gap between concentric circles of A66 A68
  measures "d149" distance between parallel lines of L42 L43
  measures "d150" radius of A71
  measures "d151" radius of A75
  measures "d152" radius of A77
  measures "d153" radius of A79
  measures "d161" diameter of A91
  measures "d162" radius of A93
  measures "d165" distance from line of A101.centre L61
  measures "d169" diameter of A105
  measures "d180" diameter of A106
extrude "Выдавливание13" add sketch "Эскиз9" along normal blind 6 contours A75 A88 L49 L46 L55 A79 A4 | A73 A72 L45 A71 A80 A74 A88 | A74 A80 A77 L49 A88 | L53 A82 A83 A89 L52 A85 A87 A81 | A84 A90 A86 L56 L51 L52 A89
extrude "Выдавливание14" add sketch "Эскиз9" along normal blind 34.8 contours A73 A72 L45 A71 A80 A74 A88 | A74 A80 A77 L49 A88 | L53 A82 A83 A89 L52 A85 A87 A81
ref_plane "РабПлоскость3" through (23.5, 10.85, -93.6349) normal (0, 0, 1) x (1, 0, 0)
sketch "Эскиз10" plane through (23.5, 10.85, -93.6349) normal (0, 0, 1) x (1, 0, 0)
  arc A0 (0, 0) -> (-2.0546, 2.8471) centre (-3, 0) ccw projected
  line L0 (-2.0546, -10.85) -> (-2.0546, 2.8471) construction
  line L1 (0, -10.85) -> (-2.0546, -10.85) construction
  line L2 (0, -10.85) -> (0, 0) construction
  spline S0 degree 4 poles (-4.4081, 2.9941) (-4.3815, 2.997) (-4.3546, 2.999) (-4.3274, 3) (-4.3, 3) knots 0 0 0 0 0 1 1 1 1 1 projected
  line L3 (-4.4081, -1.0919) -> (-4.4081, 2.9941) construction
  line L4 (-3.5, -2) -> (-4.4081, -1.0919) projected
  line L5 (-3.5, -7) -> (-3.5, -2) construction
  line L6 (-4.4081, -7) -> (-3.5, -7) construction
  line L7 (-4.4081, -10.85) -> (-4.4081, -7) construction
  line L8 (-2.0546, -10.85) -> (-4.4081, -10.85) construction
  line L9 (-2.0546, 2.8471) -> (-2.0546, -10.85) construction
  spline S1 degree 6 poles (-3, 3) (-2.9139, 3) (-2.8267, 2.997) (-2.7386, 2.991) (-2.6499, 2.9817) (-2.5611, 2.9691) (-2.4019, 2.9407) (-2.3314, 2.926) (-2.2612, 2.9092) (-2.1915, 2.8904) (-2.1226, 2.8697) (-2.0546, 2.8471) knots 0 0 0 0 0 0 0 0.556009 0.556009 0.556009 0.556009 0.556009 1 1 1 1 1 1 1 projected
  line L10 (-4.3, 3) -> (-3, 3) projected
  arc A1 (-4.4081, 2.9941) -> (-5.3, 2) centre (-4.3, 2) ccw projected
  line L11 (-5.3, -0.2) -> (-5.3, 2) projected
  line L12 (-4.4081, -1.0919) -> (-5.3, -0.2) projected
  line L13 (-4.4081, -1.0919) -> (-4.4081, 2.9941) construction
  line L14 (-42.5919, -1.0919) -> (-42.5919, 2.9941) projected
  arc A2 (-41.7, 2) -> (-42.5919, 2.9941) centre (-42.7, 2) ccw projected
  line L15 (-42.5919, -1.0919) -> (-42.5919, 2.9941) projected
  line L16 (-41.7, -0.2) -> (-42.5919, -1.0919) projected
  line L17 (-41.7, -0.2) -> (-41.7, 2) projected
  spline S2 degree 7 poles (-42.7, 3) (-42.6843, 3) (-42.6687, 2.9997) (-42.6532, 2.9991) (-42.6378, 2.9983) (-42.6224, 2.9972) (-42.6071, 2.9958) (-42.5919, 2.9941) knots 0 0 0 0 0 0 0 0 1 1 1 1 1 1 1 1 projected
  line L18 (-44, 3) -> (-42.7, 3) projected
  spline S3 degree 5 poles (-44.9454, 2.8471) (-44.8643, 2.8741) (-44.782, 2.8982) (-44.6986, 2.9194) (-44.6145, 2.9376) (-44.4235, 2.9719) (-44.3163, 2.9862) (-44.2095, 2.9955) (-44.1039, 3) (-44, 3) knots 0 0 0 0 0 0 0.440959 0.440959 0.440959 0.440959 1 1 1 1 1 1 projected
  line L19 (-44.9454, -10.85) -> (-44.9454, 2.8471) construction
  line L20 (-42.5919, -10.85) -> (-44.9454, -10.85) construction
  line L21 (-42.5919, -10.85) -> (-42.5919, -7) construction
  line L22 (-43.5, -7) -> (-42.5919, -7) construction
  line L23 (-43.5, -7) -> (-43.5, -2) construction
  line L24 (-42.5919, -1.0919) -> (-43.5, -2) projected
  line L25 (-42.5919, -1.0919) -> (-42.5919, 2.9941) projected
  arc A3 (-44.9454, 2.8471) -> (-47, 0) centre (-44, 0) ccw projected
  line L26 (-47, -10.85) -> (-47, 0) construction
  line L27 (-44.9454, -10.85) -> (-47, -10.85) construction
  line L28 (-44.9454, -10.85) -> (-44.9454, 2.8471) construction
  line L29 (6.6851, -2.85) -> (-3.5, -2.85) construction
  line L30 (-3.0402, -2.85) -> (-3.5, -2.85) construction
  line L31 (0, -2.85) -> (-3.0402, -2.85) construction
  line L32 (0, -2.85) -> (1.5, -2.85) construction
  line L33 (1.5, -2.85) -> (3.522, -2.85) construction
  line L34 (3.522, -2.85) -> (6.6851, -2.85) construction
  line L35 (-43.5, -2.85) -> (-53.6851, -2.85) construction
  line L36 (-53.6851, -2.85) -> (-50.522, -2.85) construction
  line L37 (-50.522, -2.85) -> (-48.5, -2.85) construction
  line L38 (-48.5, -2.85) -> (-47, -2.85) construction
  line L39 (-43.9598, -2.85) -> (-47, -2.85) construction
  line L40 (-43.5, -2.85) -> (-43.9598, -2.85) construction
  line L41 (0, -10.85) -> (0, 0) projected
  line L42 (0, -2.85) -> (0, 0)
  line L43 (-3.5, -7) -> (-3.5, -2) projected
  line L44 (-3.5, -2.85) -> (-3.5, -2)
  line L45 (0, -2.85) -> (-3.5, -2.85)
  line L46 (-42.5919, -1.0919) -> (-43.5, -2) projected
  line L47 (-43.5, -2) -> (-43.5, -2.85)
  line L48 (-43.5, -7) -> (-43.5, -2) projected
  line L49 (-43.5, -2.85) -> (-47, -2.85)
  line L50 (-47, -10.85) -> (-47, 0) projected
  line L51 (-47, -2.85) -> (-47, 0)
  point P0 (-23.5, -10.85)
  point P1 (-44.9454, 2.8471)
  point P2 (-4.4081, -1.0919)
  point P3 (-2.0546, 2.8471)
  point P4 (-4.4081, 2.9941)
  point P5 (0, -2)
  point P6 (-47, -2)
  point P7 (-47, -2)
  point P8 (0, -2)
  constraints: 12 end point, 5 collinear, 1 perpendicular, 4 other
extrude "Выдавливание15" add sketch "Эскиз10" against normal blind 5.5
extrude "Выдавливание16" add sketch "Эскиз9" along normal up to surface (1.85 mm away) contours L59 A106 A91 | A91 L59 A96 A97 A95 | A92 A93 L59 A106 | L59 A94 A92 | A95 A97 A96 L62 L61 L60
sketch "Эскиз11" plane through (0, 0, 0) normal (0, -1, 0) x (1, 0, 0)
  arc A0 (1.5944, -46.1335) -> (-1.5944, -46.1335) centre (0, -46) ccw projected
  circle A1 centre (24, -98.1071) radius 1.6 projected
  circle A2 centre (-24, -98.1071) radius 1.6 projected
  point P0 (0, 0)
extrude "Выдавливание17" cut sketch "Эскиз11" against normal up to surface (8 mm away)
ref_plane "РабПлоскость10" through (0, 36.5, 0) normal (0, 1, 0) x (1, 0, 0)